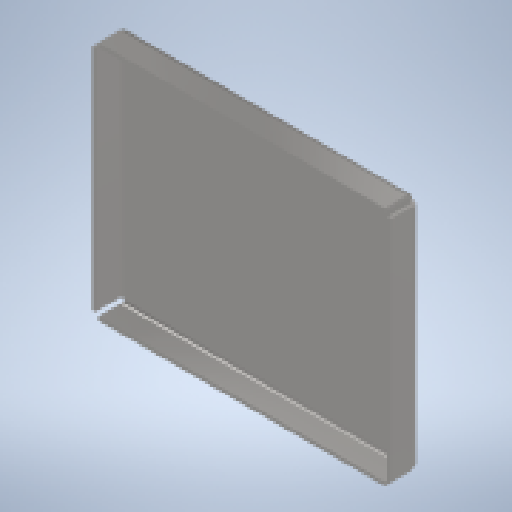
# Autodesk Inventor part: FrameBase
Saved by Autodesk Inventor 2024 (Build 280153000, 153)
## iProperties
Created: 2024-09-07
Part Number: FrameBase
Material: Stainless Steel
Document SubType Name: Sheet Metal
Designer: Tommy Rohmann
Density: 8 g/cm^3
Sheet Metal Rule: 1/8 SS Sheet
Appearance: Semi-Polished
Author: Tommy Rohmann
Autodesk Inventor part; units mm, degrees
note: some values were not read from the file. Chosen so that the rebuilt part matches the saved one: corner form of "Plate2".
ref_plane "YZ Plane" through (0, 0, 0) normal (1, 0, 0) x (0, 1, 0)
ref_plane "XZ Plane" through (0, 0, 0) normal (0, 1, 0) x (-1, 0, 0)
ref_plane "XY Plane" through (0, 0, 0) normal (0, 0, 1) x (1, 0, 0)
sketch "Sketch1" plane through (0, 0, 0) normal (0, 0, 1) x (1, 0, 0)
  line L0 (130.175, -104.775) -> (-130.175, -104.775)
  line L1 (-130.175, -104.775) -> (-130.175, 104.775)
  line L2 (-130.175, 104.775) -> (130.175, 104.775)
  line L3 (130.175, 104.775) -> (130.175, -104.775)
  line L4 (130.175, -104.775) -> (-130.175, 104.775) construction
  line L5 (-130.175, -104.775) -> (130.175, 104.775) construction
  point P0 (0, 0)
  dimension "d0" = 260.35
  dimension "d1" = 209.55
  measures "d0" distance of L1.end L2.end
  measures "d1" distance of L0.end L1.end
extrude "Plate1" add sketch "Sketch1" along normal blind 3.175
sketch "Sketch2" plane through (130.175, -101.6, 0) normal (0, -1, 0) x (1, 0, 0)
  line L0 (-260.35, 0) -> (0, 0)
  line L1 (0, 0) -> (0, 25.4)
  line L2 (0, 25.4) -> (-260.35, 25.4)
  line L3 (-260.35, 25.4) -> (-260.35, 0)
  constraints: 6 end point, 1 horizontal, 1 perpendicular, 1 vertical
edge flange "Flange1" height 25.4 angle 90 thickness 3.175 bend radius 3.175 thickness toward (0, -1, 0) relief tear relief width 3.175 relief depth 1.5875 corner gap 3.175 corner form 2 edges at (0, -104.775, 3.175) (130.175, 0, 3.175) (0, 104.775, 3.175) (-130.175, 0, 3.175) wall of the first edge with corners at (-130.175, -101.6, 0) (130.175, -101.6, 0) (130.175, -101.6, 25.4) (-130.175, -101.6, 25.4)
bend "Bend1"
corner "Corner1"
equation "\"d0\" = MachineMaxLength - 2 * Thickness"
equation "\"d1\" = MachineMaxWidth - 2 * Thickness"
equation "\"d2\" = Thickness"
equation "\"d3\" = BendReliefWidth"
equation "\"d4\" = BendReliefDepth"
equation "\"d5\" = MinimumRemnant"
equation "\"d6\" = TransitionRadius"
equation "\"d9\" = BendRadius"
equation "\"d10\" = CornerReliefSize"
equation "\"d11\" = GapSize"
equation "\"d12\" = JacobiRadiusSize"
equation "\"BendRadius\" = Thickness"
equation "\"BendReliefWidth\" = Thickness"
equation "\"BendReliefDepth\" = 0.5 * Thickness"
equation "\"CornerReliefSize\" = 4 * Thickness"
equation "\"MinimumRemnant\" = 2 * Thickness"
equation "\"TransitionRadius\" = BendRadius"
equation "\"JacobiRadiusSize\" = BendRadius"
equation "\"GapSize\" = Thickness"
equation "\"MachineMaxHeight\" = 539.75"
equation "\"MachineMaxWidth\" = 215.9"
equation "\"MachineMaxLength\" = 266.7"
equation "\"MachineFluidCapacity\" = 25.4"
equation "\"MaxCompressiveCapacity\" = 20320"
equation "\"WashChamberOD\" = 114.3"
equation "\"WashChamberID\" = 101.6"
equation "\"ConduitThickness\" = 152.4"
equation "\"SealedSurfaceOffset\" = 0.15875"
equation "\"StaticORingThickness\" = 4.7625"
equation "\"Thickness\" = 3.175"
body "Solid1"
